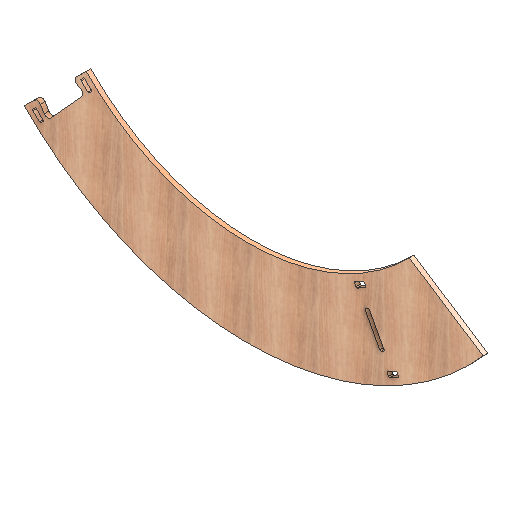
# Autodesk Inventor part: Platform C4
Saved by Autodesk Inventor 2021 (Build 250183000, 183)
## iProperties
Created: 2020-05-09
Part Number: Platform C4
Material: Wood (Birch)
Document SubType Name: Modeling
Designer: Dan Wikman
Density: 0.55 g/cm^3
Appearance: Birch - Natural Polished
Mass: 5518.98 g
Surface Area: 12042.8 cm^2
Volume: 10034.5 cm^3
Autodesk Inventor part; units mm, degrees
ref_plane "YZ Plane" through (0, 0, 0) normal (1, 0, 0) x (0, 1, 0)
ref_plane "XZ Plane" through (0, 0, 0) normal (0, 1, 0) x (-1, 0, 0)
ref_plane "XY Plane" through (0, 0, 0) normal (0, 0, 1) x (1, 0, 0)
sketch "CONTOURS" plane through (0, 0, 0) normal (0, 0, 1) x (1, 0, 0)
  line L0 (29.0412, 889.8609) -> (69.6135, 929.6413)
  arc A0 (92.1865, 926.768) -> (69.6135, 929.6413) centre (79.765, 919.2877) ccw
  line L1 (92.1865, 926.768) -> (107.0781, 902.0398)
  arc A1 (107.0781, 902.0398) -> (131.8211, 899.605) centre (120.3563, 910.0361) ccw
  line L2 (131.8211, 899.605) -> (252.9238, 1032.7101)
  arc A2 (252.9238, 1032.7101) -> (248.9601, 1056.7052) centre (241.459, 1043.1412) ccw
  line L3 (248.9601, 1056.7052) -> (234.1791, 1064.8793)
  arc A3 (231.0447, 1087.9218) -> (234.1791, 1064.8793) centre (241.1963, 1077.5683) ccw
  line L4 (231.0447, 1087.9218) -> (270.3869, 1126.4961)
  arc A4 (270.3869, 1126.4961) -> (1527.2637, 1126.4961) centre (898.8253, 1743.5906) ccw
  line L5 (1527.2637, 1126.4961) -> (1815.1018, 939.9773)
  arc A5 (29.0412, 889.8609) -> (1815.1018, 939.9773) centre (898.8169, 1743.6721) ccw
  constraints: 12 end point, 12 point on circle, 6 centre point
sketch "HOLES" plane through (0, 0, 0) normal (0, 0, 1) x (1, 0, 0)
  line L0 (290.0252, 1067.7256) -> (282.3828, 1059.8139)
  arc A0 (276.7268, 1059.716) -> (282.3828, 1059.8139) centre (279.5059, 1062.593) ccw
  line L1 (276.7268, 1059.716) -> (250.8342, 1084.7274)
  arc A1 (250.7363, 1090.3834) -> (250.8342, 1084.7274) centre (253.6132, 1087.6044) ccw
  line L2 (250.7363, 1090.3834) -> (258.3786, 1098.2951)
  arc A2 (264.0347, 1098.393) -> (258.3786, 1098.2951) centre (261.2556, 1095.516) ccw
  line L3 (264.0347, 1098.393) -> (289.9273, 1073.3816)
  arc A3 (290.0252, 1067.7256) -> (289.9273, 1073.3816) centre (287.1482, 1070.5046) ccw
  line L4 (102.1615, 873.2431) -> (94.5191, 865.3315)
  arc A4 (88.8631, 865.2335) -> (94.5191, 865.3315) centre (91.6422, 868.1105) ccw
  line L5 (88.8631, 865.2335) -> (62.9705, 890.245)
  arc A5 (62.8726, 895.901) -> (62.9705, 890.245) centre (65.7496, 893.1219) ccw
  line L6 (62.8726, 895.901) -> (70.515, 903.8126)
  arc A6 (76.171, 903.9105) -> (70.515, 903.8126) centre (73.3919, 901.0336) ccw
  arc A7 (102.1615, 873.2431) -> (102.0636, 878.8991) centre (99.2846, 876.0221) ccw
  line L7 (1358.4331, 945.869) -> (1353.2703, 955.5821)
  arc A8 (1353.2703, 955.5821) -> (1347.8609, 957.2368) centre (1349.7382, 953.7047) ccw
  line L8 (1347.8609, 957.2368) -> (1316.0723, 940.3404)
  arc A9 (1316.0723, 940.3404) -> (1314.4176, 934.931) centre (1317.9497, 936.8084) ccw
  line L9 (1314.4176, 934.931) -> (1319.5804, 925.2178)
  arc A10 (1319.5804, 925.2178) -> (1324.9899, 923.5631) centre (1323.1125, 927.0952) ccw
  line L10 (1324.9899, 923.5631) -> (1356.7784, 940.4595)
  arc A11 (1356.7784, 940.4595) -> (1358.4331, 945.869) centre (1354.901, 943.9916) ccw
  line L11 (1441.3284, 696.1636) -> (1446.4912, 686.4505)
  arc A12 (1446.4912, 686.4505) -> (1451.9006, 684.7958) centre (1450.0232, 688.3278) ccw
  line L12 (1451.9006, 684.7958) -> (1483.6892, 701.6922)
  arc A13 (1483.6892, 701.6922) -> (1485.3438, 707.1016) centre (1481.8118, 705.2242) ccw
  line L13 (1485.3438, 707.1016) -> (1480.181, 716.8148)
  arc A14 (1480.181, 716.8148) -> (1474.7716, 718.4695) centre (1476.649, 714.9374) ccw
  line L14 (1474.7716, 718.4695) -> (1442.9831, 701.5731)
  arc A15 (1442.9831, 701.5731) -> (1441.3284, 696.1636) centre (1444.8604, 698.041) ccw
  line L15 (1363.2554, 875.1779) -> (1357.078, 871.8854)
  arc A16 (1357.078, 871.8854) -> (1355.4295, 866.4741) centre (1358.9594, 868.3555) ccw
  line L16 (1355.4295, 866.4741) -> (1412.8118, 758.8114)
  arc A17 (1412.8118, 758.8114) -> (1418.2231, 757.1628) centre (1416.3417, 760.6927) ccw
  line L17 (1418.2231, 757.1628) -> (1427.9304, 762.3366)
  arc A18 (1427.9304, 762.3366) -> (1429.579, 767.7479) centre (1426.049, 765.8666) ccw
  line L18 (1429.579, 767.7479) -> (1372.1967, 875.4107)
  arc A19 (1372.1967, 875.4107) -> (1366.7853, 877.0592) centre (1368.6667, 873.5293) ccw
  line L19 (1366.7853, 877.0592) -> (1363.2554, 875.1779)
  line L20 (76.171, 903.9105) -> (102.0636, 878.8991)
  constraints: 42 end point, 40 point on circle, 20 centre point
sketch "LETTERS" plane through (0, 0, 0) normal (0, 0, 1) x (1, 0, 0)
  line L0 (246.1168, 901.1678) -> (246.0351, 901.3924)
  line L1 (246.0351, 901.3924) -> (245.9598, 901.6191)
  line L2 (245.9598, 901.6191) -> (245.8908, 901.8478)
  line L3 (245.8908, 901.8478) -> (245.8282, 902.0782)
  line L4 (245.8282, 902.0782) -> (245.7719, 902.3102)
  line L5 (245.7719, 902.3102) -> (245.722, 902.5436)
  line L6 (245.722, 902.5436) -> (245.6784, 902.7782)
  line L7 (245.6784, 902.7782) -> (245.6412, 903.0139)
  line L8 (245.6412, 903.0139) -> (245.6104, 903.2504)
  line L9 (245.6104, 903.2504) -> (245.586, 903.4876)
  line L10 (245.586, 903.4876) -> (245.5679, 903.7253)
  line L11 (245.5679, 903.7253) -> (245.5562, 903.9634)
  line L12 (245.5562, 903.9634) -> (245.551, 904.2015)
  line L13 (245.551, 904.2015) -> (245.5521, 904.4397)
  line L14 (245.5521, 904.4397) -> (245.5596, 904.6777)
  line L15 (245.5596, 904.6777) -> (245.5736, 904.9152)
  line L16 (245.5736, 904.9152) -> (245.594, 905.1522)
  line L17 (245.594, 905.1522) -> (245.6208, 905.3885)
  line L18 (245.6208, 905.3885) -> (245.654, 905.6238)
  line L19 (245.654, 905.6238) -> (245.6937, 905.8581)
  line L20 (245.6937, 905.8581) -> (245.7398, 906.0911)
  line L21 (245.7398, 906.0911) -> (245.7923, 906.3226)
  line L22 (245.7923, 906.3226) -> (245.8513, 906.5525)
  line L23 (245.8513, 906.5525) -> (245.9168, 906.7806)
  line L24 (245.9168, 906.7806) -> (245.9887, 907.0067)
  line L25 (245.9887, 907.0067) -> (246.0671, 907.2306)
  line L26 (246.0671, 907.2306) -> (246.1519, 907.4522)
  line L27 (246.1519, 907.4522) -> (246.2433, 907.6712)
  line L28 (246.2433, 907.6712) -> (246.3411, 907.8876)
  line L29 (246.3411, 907.8876) -> (246.4454, 908.1011)
  line L30 (246.4454, 908.1011) -> (246.5562, 908.3115)
  line L31 (246.5562, 908.3115) -> (246.6735, 908.5187)
  line L32 (246.6735, 908.5187) -> (246.7973, 908.7225)
  line L33 (246.7973, 908.7225) -> (246.9274, 908.9228)
  line L34 (246.9274, 908.9228) -> (247.0637, 909.1194)
  line L35 (247.0637, 909.1194) -> (247.2058, 909.3123)
  line L36 (247.2058, 909.3123) -> (247.3538, 909.5013)
  line L37 (247.3538, 909.5013) -> (247.5073, 909.6863)
  line L38 (247.5073, 909.6863) -> (247.6661, 909.8672)
  line L39 (247.6661, 909.8672) -> (247.8302, 910.0439)
  line L40 (247.8302, 910.0439) -> (247.9992, 910.2163)
  line L41 (247.9992, 910.2163) -> (248.1731, 910.3842)
  line L42 (248.1731, 910.3842) -> (248.3515, 910.5476)
  line L43 (248.3515, 910.5476) -> (248.5344, 910.7063)
  line L44 (248.5344, 910.7063) -> (248.7216, 910.8603)
  line L45 (248.7216, 910.8603) -> (248.9128, 911.0093)
  line L46 (248.9128, 911.0093) -> (249.1078, 911.1534)
  line L47 (249.1078, 911.1534) -> (249.3066, 911.2923)
  line L48 (249.3066, 911.2923) -> (249.5088, 911.426)
  line L49 (249.5088, 911.426) -> (249.7143, 911.5543)
  line L50 (249.7143, 911.5543) -> (249.9229, 911.6772)
  line L51 (249.9229, 911.6772) -> (250.1344, 911.7944)
  line L52 (250.1344, 911.7944) -> (250.3487, 911.906)
  line L53 (250.3487, 911.906) -> (250.5655, 912.0118)
  line L54 (250.5655, 912.0118) -> (250.7846, 912.1117)
  line L55 (250.7846, 912.1117) -> (251.0059, 912.2055)
  line L56 (251.0059, 912.2055) -> (251.2292, 912.2932)
  line L57 (251.2292, 912.2932) -> (251.4543, 912.3746)
  line L58 (251.4543, 912.3746) -> (251.6809, 912.4497)
  line L59 (251.6809, 912.4497) -> (251.909, 912.5182)
  line L60 (251.909, 912.5182) -> (252.1383, 912.5802)
  line L61 (252.1383, 912.5802) -> (252.3686, 912.6354)
  line L62 (252.3686, 912.6354) -> (252.5997, 912.6838)
  line L63 (252.5997, 912.6838) -> (252.8315, 912.7253)
  line L64 (252.8315, 912.7253) -> (253.0638, 912.7597)
  line L65 (253.0638, 912.7597) -> (253.2964, 912.7872)
  line L66 (253.2964, 912.7872) -> (253.5293, 912.8077)
  line L67 (253.5293, 912.8077) -> (253.7624, 912.8215)
  line L68 (253.7624, 912.8215) -> (253.9954, 912.8287)
  line L69 (253.9954, 912.8287) -> (254.2285, 912.8292)
  line L70 (254.2285, 912.8292) -> (254.4614, 912.8232)
  line L71 (254.4614, 912.8232) -> (254.694, 912.8108)
  line L72 (254.694, 912.8108) -> (254.9262, 912.7921)
  line L73 (254.9262, 912.7921) -> (255.158, 912.7672)
  line L74 (255.158, 912.7672) -> (255.3893, 912.7361)
  line L75 (255.3893, 912.7361) -> (255.6198, 912.699)
  line L76 (255.6198, 912.699) -> (255.8496, 912.656)
  line L77 (255.8496, 912.656) -> (256.0785, 912.6071)
  line L78 (256.0785, 912.6071) -> (256.3065, 912.5524)
  line L79 (256.3065, 912.5524) -> (256.5333, 912.4921)
  line L80 (256.5333, 912.4921) -> (256.759, 912.4263)
  line L81 (256.759, 912.4263) -> (256.9834, 912.3549)
  line L82 (256.9834, 912.3549) -> (257.2064, 912.2781)
  line L83 (257.2064, 912.2781) -> (257.4279, 912.1961)
  line L84 (257.4279, 912.1961) -> (257.6478, 912.1088)
  line L85 (257.6478, 912.1088) -> (257.8661, 912.0165)
  line L86 (257.8661, 912.0165) -> (258.0825, 911.9191)
  line L87 (258.0825, 911.9191) -> (258.297, 911.8168)
  line L88 (258.297, 911.8168) -> (258.5095, 911.7097)
  line L89 (258.5095, 911.7097) -> (258.7199, 911.5978)
  line L90 (258.7199, 911.5978) -> (258.9281, 911.4814)
  line L91 (258.9281, 911.4814) -> (259.134, 911.3603)
  line L92 (259.134, 911.3603) -> (259.3375, 911.2348)
  line L93 (259.3375, 911.2348) -> (259.5384, 911.105)
  line L94 (259.5384, 911.105) -> (259.7367, 910.9709)
  line L95 (259.7367, 910.9709) -> (259.9323, 910.8326)
  line L96 (259.9323, 910.8326) -> (260.1251, 910.6902)
  line L97 (260.1251, 910.6902) -> (260.315, 910.5438)
  line L98 (260.315, 910.5438) -> (260.5019, 910.3936)
  line L99 (260.5019, 910.3936) -> (260.6858, 910.2394)
  line L100 (260.6858, 910.2394) -> (260.8666, 910.0816)
  line L101 (260.8666, 910.0816) -> (261.0443, 909.92)
  line L102 (261.0443, 909.92) -> (261.2187, 909.7549)
  line L103 (261.2187, 909.7549) -> (261.3897, 909.5863)
  line L104 (261.3897, 909.5863) -> (261.5574, 909.4142)
  line L105 (261.5574, 909.4142) -> (261.7217, 909.2389)
  line L106 (261.7217, 909.2389) -> (261.8825, 909.0602)
  line L107 (261.8825, 909.0602) -> (262.0396, 908.8784)
  line L108 (262.0396, 908.8784) -> (262.1932, 908.6935)
  line L109 (262.1932, 908.6935) -> (262.343, 908.5056)
  line L110 (262.343, 908.5056) -> (262.489, 908.3148)
  line L111 (262.489, 908.3148) -> (262.6311, 908.1211)
  line L112 (262.6311, 908.1211) -> (262.7694, 907.9247)
  line L113 (262.7694, 907.9247) -> (262.9036, 907.7256)
  line L114 (262.9036, 907.7256) -> (263.0338, 907.5239)
  line L115 (263.0338, 907.5239) -> (263.1599, 907.3197)
  line L116 (263.1599, 907.3197) -> (263.2817, 907.1131)
  line L117 (263.2817, 907.1131) -> (263.3993, 906.9041)
  line L118 (263.3993, 906.9041) -> (263.5126, 906.6929)
  line L119 (263.5126, 906.6929) -> (263.6214, 906.4795)
  line L120 (263.6214, 906.4795) -> (263.7258, 906.264)
  line L121 (263.7258, 906.264) -> (263.8257, 906.0465)
  line L122 (263.8257, 906.0465) -> (263.9209, 905.827)
  line L123 (263.9209, 905.827) -> (264.0114, 905.6057)
  line L124 (264.0114, 905.6057) -> (264.0973, 905.3826)
  line L125 (264.0973, 905.3826) -> (264.1782, 905.1579)
  line L126 (264.1782, 905.1579) -> (264.2544, 904.9316)
  line L127 (264.2544, 904.9316) -> (264.3255, 904.7037)
  line L128 (264.3255, 904.7037) -> (264.3917, 904.4744)
  line L129 (264.3917, 904.4744) -> (264.4527, 904.2438)
  line L130 (264.4527, 904.2438) -> (264.5087, 904.012)
  line L131 (264.5087, 904.012) -> (264.5596, 903.7792)
  line L132 (264.5596, 903.7792) -> (264.6053, 903.5455)
  line L133 (264.6053, 903.5455) -> (264.6458, 903.3109)
  line L134 (264.6458, 903.3109) -> (264.6811, 903.0757)
  line L135 (264.6811, 903.0757) -> (264.7111, 902.84)
  line L136 (264.7111, 902.84) -> (264.7358, 902.6039)
  line L137 (264.7358, 902.6039) -> (264.7552, 902.3675)
  line L138 (264.7552, 902.3675) -> (264.7692, 902.1309)
  line L139 (264.7692, 902.1309) -> (264.7779, 901.8943)
  line L140 (264.7779, 901.8943) -> (264.781, 901.6578)
  line L141 (264.781, 901.6578) -> (264.7787, 901.4216)
  line L142 (264.7787, 901.4216) -> (264.7709, 901.1857)
  line L143 (264.7709, 901.1857) -> (264.7576, 900.9503)
  line L144 (264.7576, 900.9503) -> (264.7387, 900.7155)
  line L145 (264.7387, 900.7155) -> (264.7141, 900.4815)
  line L146 (264.7141, 900.4815) -> (264.684, 900.2483)
  line L147 (264.684, 900.2483) -> (264.6481, 900.0162)
  line L148 (264.6481, 900.0162) -> (264.6065, 899.7851)
  line L149 (264.6065, 899.7851) -> (264.5592, 899.5554)
  line L150 (264.5592, 899.5554) -> (264.5061, 899.327)
  line L151 (264.5061, 899.327) -> (264.4472, 899.1002)
  line L152 (264.4472, 899.1002) -> (264.3824, 898.875)
  line L153 (264.3824, 898.875) -> (264.3117, 898.6515)
  line L154 (264.3117, 898.6515) -> (264.2351, 898.43)
  line L155 (264.2351, 898.43) -> (264.1526, 898.2105)
  line L156 (264.1526, 898.2105) -> (264.064, 897.9932)
  line L157 (264.064, 897.9932) -> (263.9694, 897.7781)
  line L158 (263.9694, 897.7781) -> (263.8688, 897.5655)
  line L159 (263.8688, 897.5655) -> (263.762, 897.3554)
  line L160 (263.6492, 897.148) -> (263.5303, 896.9434)
  line L161 (263.5303, 896.9434) -> (263.4056, 896.7417)
  line L162 (263.4056, 896.7417) -> (263.2753, 896.5431)
  line L163 (263.2753, 896.5431) -> (263.1393, 896.3477)
  line L164 (263.1393, 896.3477) -> (262.9979, 896.1557)
  line L165 (262.9979, 896.1557) -> (262.8513, 895.9671)
  line L166 (262.8513, 895.9671) -> (262.6996, 895.7821)
  line L167 (262.6996, 895.7821) -> (262.5428, 895.6009)
  line L168 (262.5428, 895.6009) -> (262.3813, 895.4235)
  line L169 (262.3813, 895.4235) -> (262.215, 895.2501)
  line L170 (262.215, 895.2501) -> (262.0442, 895.0809)
  line L171 (262.0442, 895.0809) -> (261.869, 894.9159)
  line L172 (261.869, 894.9159) -> (261.6896, 894.7553)
  line L173 (261.6896, 894.7553) -> (261.506, 894.5993)
  line L174 (261.506, 894.5993) -> (261.3185, 894.4479)
  line L175 (261.3185, 894.4479) -> (261.1271, 894.3014)
  line L176 (261.1271, 894.3014) -> (260.9321, 894.1597)
  line L177 (260.9321, 894.1597) -> (260.7336, 894.0231)
  line L178 (260.7336, 894.0231) -> (260.5316, 893.8917)
  line L179 (260.5316, 893.8917) -> (260.3264, 893.7657)
  line L180 (260.3264, 893.7657) -> (260.1181, 893.6451)
  line L181 (260.1181, 893.6451) -> (259.9069, 893.5301)
  line L182 (259.9069, 893.5301) -> (259.6928, 893.4208)
  line L183 (259.6928, 893.4208) -> (259.4761, 893.3174)
  line L184 (259.4761, 893.3174) -> (259.2568, 893.22)
  line L185 (259.2568, 893.22) -> (259.0352, 893.1287)
  line L186 (259.0352, 893.1287) -> (258.8114, 893.0437)
  line L187 (258.8114, 893.0437) -> (258.5854, 892.965)
  line L188 (258.5854, 892.965) -> (258.3575, 892.8929)
  line L189 (258.3575, 892.8929) -> (258.1278, 892.8275)
  line L190 (258.1278, 892.8275) -> (257.8965, 892.7688)
  line L191 (257.8965, 892.7688) -> (257.6637, 892.717)
  line L192 (257.6637, 892.717) -> (257.4295, 892.6722)
  line L193 (257.4295, 892.6722) -> (257.1943, 892.6343)
  line L194 (257.1943, 892.6343) -> (256.9581, 892.6033)
  line L195 (256.9581, 892.6033) -> (256.7213, 892.5793)
  line L196 (256.7213, 892.5793) -> (256.484, 892.5622)
  line L197 (256.484, 892.5622) -> (256.2464, 892.552)
  line L198 (256.2464, 892.552) -> (256.0087, 892.5488)
  line L199 (256.0087, 892.5488) -> (255.7711, 892.5526)
  line L200 (255.7711, 892.5526) -> (255.5339, 892.5633)
  line L201 (255.5339, 892.5633) -> (255.2972, 892.5809)
  line L202 (255.2972, 892.5809) -> (255.0612, 892.6055)
  line L203 (255.0612, 892.6055) -> (254.8262, 892.6371)
  line L204 (254.8262, 892.6371) -> (254.5924, 892.6756)
  line L205 (254.5924, 892.6756) -> (254.3599, 892.721)
  line L206 (254.3599, 892.721) -> (254.1289, 892.7734)
  line L207 (254.1289, 892.7734) -> (253.8997, 892.8328)
  line L208 (253.8997, 892.8328) -> (253.6725, 892.8992)
  line L209 (253.6725, 892.8992) -> (253.4474, 892.9725)
  line L210 (253.4474, 892.9725) -> (253.2248, 893.0528)
  line L211 (253.2248, 893.0528) -> (253.0047, 893.14)
  line L212 (253.0047, 893.14) -> (252.7873, 893.2342)
  line L213 (252.7873, 893.2342) -> (252.573, 893.3354)
  line L214 (252.573, 893.3354) -> (252.3619, 893.4436)
  line L215 (252.3619, 893.4436) -> (252.1541, 893.5587)
  line L216 (252.1541, 893.5587) -> (251.95, 893.6809)
  line L217 (251.95, 893.6809) -> (251.7497, 893.81)
  line L218 (251.7497, 893.81) -> (251.5533, 893.9461)
  line L219 (251.5533, 893.9461) -> (251.3612, 894.0891)
  line L220 (251.3612, 894.0891) -> (251.1734, 894.2391)
  line L221 (251.1734, 894.2391) -> (250.9903, 894.3962)
  line L222 (250.9903, 894.3962) -> (250.9005, 894.4773)
  line L223 (250.9005, 894.4773) -> (250.812, 894.5602)
  line L224 (263.762, 897.3554) -> (263.6492, 897.148)
  constraints: 450 end point, 5 perpendicular
extrude "Extrusion3" add sketch "CONTOURS" along normal blind 18
extrude "Extrusion4" cut sketch "HOLES" along normal blind 18
body "Solid2"
